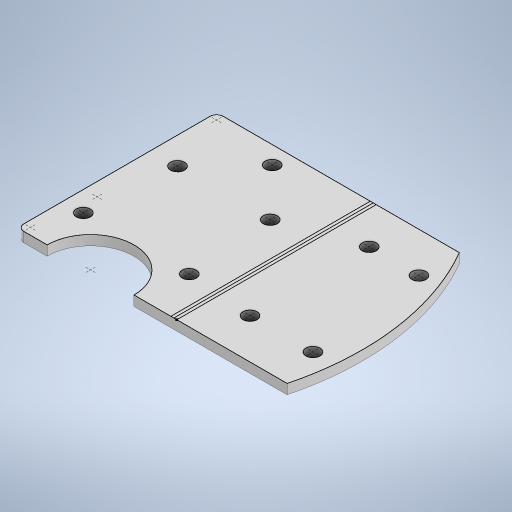
# Autodesk Inventor part: axis_2_bottom_L_frame(top)
Saved by Autodesk Inventor 2024.2 (Build 282272000, 272)
## iProperties
Created: 2024-01-11
Part Number: axis_2_bottom_L_frame(top)
Material: Generic
Document SubType Name: Modeling
Designer: chanh
Density: 1 g/cm^3
Appearance: Default
Author: chanh
Autodesk Inventor part; units mm, degrees
ref_plane "YZ Plane" through (0, 0, 0) normal (1, 0, 0) x (0, 1, 0)
ref_plane "XZ Plane" through (0, 0, 0) normal (0, 1, 0) x (-1, 0, 0)
ref_plane "XY Plane" through (0, 0, 0) normal (0, 0, 1) x (1, 0, 0)
sketch "Sketch1" plane through (0, 0, 0) normal (0, 1, 0) x (-1, 0, 0)
  line L0 (-63.7289, -30.1) -> (-63.7289, 0)
  circle A0 centre (-78.6786, -6.05) radius 1.05
  circle A1 centre (-76.6786, -24.05) radius 1.05
  circle A2 centre (-69.1786, -24.05) radius 1.05
  circle A3 centre (-69.1786, -6.05) radius 1.05
  circle A4 centre (-43.1593, -6.9) radius 1.05
  circle A5 centre (-44.1593, -20.12) radius 1.05
  circle A6 centre (-51.1593, -27.42) radius 1.05
  circle A7 centre (-58.1593, -20.12) radius 1.05
  circle A8 centre (-59.1593, -6.9) radius 1.05
  arc A9 (-40.0893, -1) -> (-41.0893, 0) centre (-41.0893, -1) ccw
  line L1 (-40.0893, -29.1) -> (-40.0893, -1)
  arc A10 (-41.0893, -30.1) -> (-40.0893, -29.1) centre (-41.0893, -29.1) ccw
  arc A11 (-80.8355, 0) -> (-76.7307, -30.1) centre (-42.1186, -10.05) ccw
  line L2 (-57.7093, 0) -> (-80.8355, 0)
  line L3 (-76.7307, -30.1) -> (-41.0893, -30.1)
  arc A12 (-57.7093, 0) -> (-44.6093, 0) centre (-51.1593, 0) ccw
  line L4 (-41.0893, 0) -> (-44.6093, 0)
  line L5 (-63.2793, -30.1) -> (-63.2793, 0)
  line L6 (-64.1786, 0) -> (-64.1786, -30.1)
  constraints: 14 end point, 13 centre point, 8 point on circle, 6 point on line, 4 vertical, 3 horizontal, 41 other
extrude "Extrusion1" add sketch "Sketch1" against normal blind 1.5
body "Solid1"
